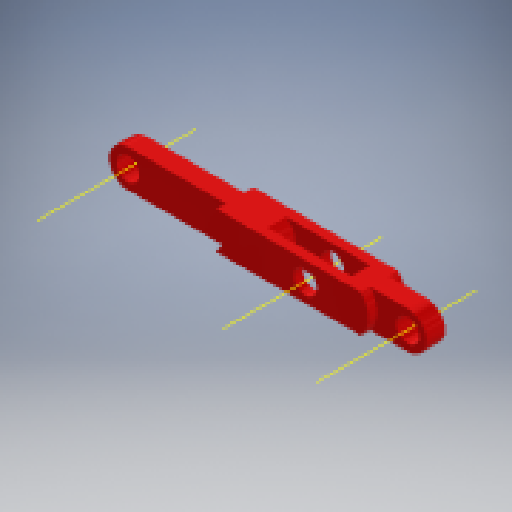
# Autodesk Inventor part: link7
Saved by Autodesk Inventor 2024.1 (Build 281209000, 209)
## iProperties
Created: 2023-09-09
Part Number: link7
Material: Aluminum 6061
Document SubType Name: Modeling
Designer: Camilo
Density: 2.7 g/cm^3
Appearance: Aluminum - Flat
Mass: 0.828529 g
Surface Area: 5.52996 cm^2
Volume: 0.306863 cm^3
Author: Camilo
Autodesk Inventor part; units mm, degrees
ref_plane "YZ Plane" through (0, 0, 0) normal (1, 0, 0) x (0, 1, 0)
ref_plane "XZ Plane" through (0, 0, 0) normal (0, 1, 0) x (-1, 0, 0)
ref_plane "XY Plane" through (0, 0, 0) normal (0, 0, 1) x (1, 0, 0)
sketch "Sketch1" plane through (0, 0, 0) normal (0, 0, 1) x (1, 0, 0)
  line L0 (0, 0) -> (15, 0)
  line L1 (0, 0) -> (-15, 0)
  line L2 (0, 0) -> (5, 0)
  circle A0 centre (-15, 0) radius 1.25
  circle A1 centre (15, 0) radius 1.25
  circle A2 centre (-15, 0) radius 2
  circle A3 centre (15, 0) radius 2
  line L3 (-15, 2) -> (15, 2)
  line L4 (-15, -2) -> (15, -2)
  circle A4 centre (5, 0) radius 1.25
  line L5 (-15, 2) -> (-4.5, 2)
  line L6 (-4.5, 2) -> (-4.5, -2)
  line L7 (-4.5, -2) -> (-15, -2)
  line L8 (-15, -2) -> (-15, 2)
  line L9 (15, 2) -> (12.5, 2)
  line L10 (12.5, -2) -> (15, -2)
  line L11 (15, -2) -> (15, 2)
  line L12 (15, 2) -> (14.5, 2)
  line L13 (15, -2) -> (14.5, -2)
  arc A5 (-4.5, -2) -> (-4.5, 2) centre (-6.7361, 0) ccw
  line L14 (5, 0) -> (1, 0)
  arc A6 (0, -2) -> (0, 2) centre (-1.5, 0) ccw
  line L15 (0, 2) -> (0, -2)
  line L16 (5, 2) -> (9, 2)
  line L17 (9, 2) -> (9, -2)
  line L18 (5, 0) -> (8, 0)
  arc A7 (9, 2) -> (9, -2) centre (10.5, 0) ccw
  line L19 (-15, 2) -> (-14.5, 2)
  line L20 (-15, -2) -> (-14.5, -2)
  arc A8 (-14.5, -2) -> (-14.5, 2) centre (-14.5, 0) ccw
  line L21 (9, 2) -> (11, 2)
  line L22 (9, -2) -> (11, -2)
  arc A9 (11, -2) -> (11, 2) centre (8.7639, 0) ccw
  point P0 (-4.5, 2)
  dimension "d1" = 15
  dimension "d2" = 15
  dimension "d3" = 5
  dimension "d4" = 2.5
  dimension "d6" = 2.5
  dimension "d7" = 4
  dimension "d8" = 4
  dimension "d9" = 2.5
  dimension "d10" = 10.5
  dimension "d16" = 4
  dimension "d17" = 3
  dimension "d18" = 4
  dimension "d21" = 4
  dimension "d23" = 3
  dimension "d24" = 0.5
  dimension "d25" = 0.5
  dimension "d26" = 2
  dimension "d35" = 2
  dimension "d36" = 2
  dimension "d37" = 3
  dimension "d38" = 4
  constraints: 46 end point, 16 point on circle, 14 point on line, 10 centre point, 5 coincident, 4 horizontal, 3 parallel, 2 midpoint, 2 perpendicular, 2 tangent
  measures "d1" distance of L0.start L0.end
  measures "d2" distance of L0.start L1.end
  measures "d3" distance of L0.start L2.end
  measures "d4" diameter of A0
  measures "d6" diameter of A1
  measures "d7" diameter of A2
  measures "d8" diameter of A3
  measures "d9" diameter of A4
  measures "d10" distance of L6.end L7.end
  measures "d16" distance of L3.start L4.start
  measures "d17" radius of A5
  measures "d18" distance of L14.start L14.end
  measures "d21" distance of L15.end L15.start
  measures "d23" distance of L14.start L18.end
  measures "d24" distance of L3.start L19.end
  measures "d25" distance of L7.end L20.end
  measures "d26" radius of A8
  measures "d35" distance of L16.end L21.end
  measures "d36" distance of L17.end L22.end
  measures "d37" radius of A9
  measures "d38" distance from line of L17 L2.end
extrude "Extrusion1" add sketch "Sketch1" along normal mid plane 2 contours A5 L6 L1 | L1 L6 A5 | L6 L4 A8 L1 | L1 A8 L3 L6 | A8 L4 A2 L1 | L1 A2 L3 A8 | A9 L0 A3 L4 | A2 L8 A0 L1 | L1 A0 L8 A2 | A2 L8 A0 | L3 A3 L0 A9 | A3 L11 A1 L0 | L0 A1 L11 A3 | L11 A1 A3
extrude "Extrusion2" add sketch "Sketch1" along normal mid plane 4 contours L15 A6 L0 | L15 L4 A5 L1 | L1 A5 L3 L15 | L0 A6 L15 | L17 L0 A9 L4 | A7 L0 L17 | L3 A9 L0 L17 | L17 L0 A7
extrude "Extrusion3" add sketch "Sketch1" along normal mid plane 4 contours A6 L3 A7 L0 A4 | L0 A4 A7 L4 A6
extrude "Extrusion4" cut sketch "Sketch1" along normal mid plane 2 contours A6 L3 A7 L0 A4 | L0 A4 A7 L4 A6
body "Solid1"
